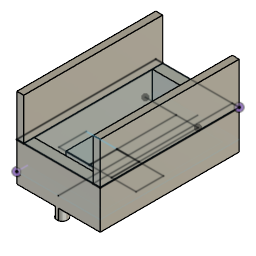
hexbug case v1 (Autodesk Fusion 360 design; units mm, degrees)
Autodesk Fusion 360 part; units mm, degrees
note: some values were not read from the file. Set by a fixed rule: which sketch regions a step uses.
sketch "Sketch1" plane through (0, 0, 0) normal (0, 0, 1) x (1, 0, 0)
  line L0 (0, 0) -> (-15.24, 0)
  line L1 (-15.24, 0) -> (-15.24, -25.4)
  line L2 (-15.24, -25.4) -> (0, -25.4)
  line L3 (0, -25.4) -> (0, 0)
  line L4 (0, 0) -> (-1.27, 0)
  line L5 (-1.27, 0) -> (-1.27, -25.4)
  line L6 (-1.27, -25.4) -> (0, -25.4)
  line L7 (0, -25.4) -> (0, 0)
  line L8 (-15.24, 0) -> (-13.97, 0)
  line L9 (-13.97, 0) -> (-13.97, -25.4)
  line L10 (-13.97, -25.4) -> (-15.24, -25.4)
  line L11 (-15.24, -25.4) -> (-15.24, 0)
  dimension "d1" = 25.4
  dimension "d2" = 15.24
  dimension "d3" = 25.4
  dimension "d4" = 1.27
  dimension "d5" = 25.4
  dimension "d6" = 1.27
  constraint horizontal L0
  constraint vertical L1
  constraint horizontal L2
  constraint vertical L3
  constraint coincident L0.start L3.end
  constraint horizontal L4
  constraint vertical L5
  constraint horizontal L6
  constraint vertical L7
  constraint horizontal L8
  constraint vertical L9
  constraint horizontal L10
  constraint vertical L11
  measures "d1" distance of L0.start L2.end
  measures "d2" distance of L0.start L0.end
  measures "d3" distance of L0.start L2.end
  measures "d4" distance of L0.start L4.end
  measures "d5" distance of L0.end L1.end
  measures "d6" distance of L0.end L8.end
extrude "Extrude1" add sketch "Sketch1" along normal blind 7.62 contours L0 L2 L3 L4 L5 L6 L7 | L0 L1 L2 L8 L9 L10 L11 makes body 1 at (0, -8.4667, 5.08) makes body 2 at (-15.24, -16.9333, 5.08)
extrude "Extrude2" add sketch "Sketch1" against normal blind 5.08 separate body makes body 3
sketch "Sketch2" plane through (0, 0, -5.08) normal (0, 0, -1) x (1, 0, 0)
  line L0 (0, 25.4) -> (-15.24, 25.4)
  line L1 (-15.24, 25.4) -> (-15.24, 0)
  line L2 (-15.24, 0) -> (0, 0)
  line L3 (0, 0) -> (0, 25.4)
  line L4 (0, 0) -> (-8.89, 0)
  line L5 (-8.89, 0) -> (-7.62, 25.4)
  line L6 (-1.143, 1.905) -> (-15.367, 1.905)
  line L7 (-15.367, 1.905) -> (-15.367, 23.495)
  line L8 (-15.367, 23.495) -> (-1.143, 23.495)
  line L9 (-1.143, 23.495) -> (-1.143, 1.905)
  line L10 (-1.143, 1.905) -> (-15.367, 23.495) construction
  line L11 (-15.367, 1.905) -> (-1.143, 23.495) construction
  point P0 (-8.255, 12.7)
  dimension "d11" = 8.89
  dimension "d12" = 21.59
  dimension "d13" = 14.224
  constraint coincident L2.end L3.start
  constraint perpendicular L1 L4
  constraint midpoint L0 L5.end
  constraint horizontal L6
  constraint perpendicular L6 L7
  constraint parallel L6 L8
  constraint parallel L7 L9
  constraint coincident L10 P0
  constraint coincident L11 P0
  constraint midpoint L5 P0
  measures "d11" distance of L2.end L4.end
  measures "d12" distance of L6.end L7.end
  measures "d13" distance of L6.start L6.end
extrude "Extrude3" cut sketch "Sketch2" against normal blind 5.08 contours L5 L6 L8 L9 | L1 L5 L6 L8 | L1 L6 L7 L8 bodies 3
sketch "Sketch3" plane through (0, 0, -5.08) normal (0, 0, -1) x (1, 0, 0)
  line L0 (-15.24, 23.495) -> (-1.143, 23.495)
  line L1 (-1.143, 23.495) -> (-1.143, 1.905)
  line L2 (-1.143, 1.905) -> (-15.24, 1.905)
  line L3 (0, 25.4) -> (-15.24, 25.4)
  line L4 (-15.24, 1.905) -> (-15.24, 0)
  line L5 (-15.24, 0) -> (0, 0)
  line L6 (0, 0) -> (0, 25.4)
  line L7 (-7.62, 0) -> (-7.62, 25.4)
  line L8 (-7.62, 12.7) -> (-9.62, 12.7)
  line L9 (-9.62, 12.7) -> (-5.62, 12.7)
  line L10 (-5.62, 12.7) -> (-5.62, 1.905)
  line L11 (-5.62, 1.905) -> (-9.62, 1.905)
  line L12 (-9.62, 1.905) -> (-9.62, 12.7)
  line L13 (-9.62, 12.7) -> (-5.62, 12.7)
  line L14 (-5.62, 12.7) -> (-5.62, 17.7)
  line L15 (-5.62, 17.7) -> (-9.62, 17.7)
  line L16 (-9.62, 17.7) -> (-9.62, 12.7)
  line L17 (-9.62, 17.7) -> (-15.24, 17.7)
  line L18 (-15.24, 17.7) -> (-15.24, 12.7)
  line L19 (-15.24, 12.7) -> (-9.62, 12.7)
  line L20 (-9.62, 12.7) -> (-9.62, 17.7)
  line L21 (-5.62, 17.7) -> (-1.143, 17.7)
  line L22 (-1.143, 17.7) -> (-1.143, 12.7)
  line L23 (-1.143, 12.7) -> (-5.62, 12.7)
  line L24 (-5.62, 12.7) -> (-5.62, 17.7)
  line L25 (-15.24, 25.4) -> (-15.24, 23.495)
  line L26 (-9.62, 1.905) -> (-15.24, 1.905)
  dimension "d16" = 2
  dimension "d17" = 4
  dimension "d18" = 5
  dimension "d19" = 4
  dimension "d32" = 5.62
  constraint midpoint L5 L7.start
  constraint midpoint L3 L7.end
  constraint midpoint L7 L8.start
  constraint perpendicular L4 L8
  constraint horizontal L9
  constraint vertical L10
  constraint horizontal L11
  constraint vertical L12
  constraint coincident L2 L10.end
  constraint horizontal L13
  constraint vertical L14
  constraint horizontal L15
  constraint vertical L16
  constraint horizontal L17
  constraint vertical L18
  constraint horizontal L19
  constraint vertical L20
  constraint horizontal L21
  constraint vertical L22
  constraint horizontal L23
  constraint vertical L24
  constraint midpoint L1 L22.end
  constraint coincident L2.end L4.start
  measures "d16" distance of L8.start L8.end
  measures "d17" distance of L10.end L11.end
  measures "d18" distance of L8.end L15.end
  measures "d19" distance of L14.end L15.end
  measures "d32" distance of L15.end L17.end
extrude "Extrude4" add sketch "Sketch3" along normal blind 2 separate body contours L7 L9 L13 L14 L15 L24 | L7 L8 L9 L13 L15 L16 L20 | L1 L14 L21 L22 L23 L24 | L2 L7 L9 L10 L11 L13 | L2 L7 L8 L9 L11 L12 L13 | L16 L17 L18 L19 L20 makes body 4
extrude "Extrude5" add 1 faces at (-5.461, -0.635, -5.08) along direction (0, 0, -1) blind 2 on bodies 3 bodies 3 4
sketch "Sketch4" plane through (0, 0, -7.08) normal (0, 0, -1) x (1, 0, 0)
  line L0 (-1.143, 17.7) -> (-15.24, 17.7)
  line L1 (-15.24, 23.495) -> (-1.143, 23.495)
  line L2 (-1.143, 23.495) -> (-1.143, 17.7)
  line L3 (-1.143, 12.7) -> (-1.143, 1.905)
  line L4 (-9.62, 1.905) -> (-15.24, 1.905)
  line L5 (-5.62, 1.905) -> (-5.62, 12.7)
  line L6 (-5.62, 12.7) -> (-1.143, 12.7)
  line L7 (0, 25.4) -> (-15.24, 25.4)
  line L8 (-15.24, 1.905) -> (-15.24, 0)
  line L9 (-15.24, 0) -> (0, 0)
  line L10 (0, 0) -> (0, 25.4)
  line L11 (-15.24, 12.7) -> (-9.62, 12.7)
  line L12 (-9.62, 12.7) -> (-9.62, 1.905)
  line L13 (-7.62, 0) -> (-7.62, 25.4)
  line L14 (-5.62, 0) -> (-5.62, 1.905)
  line L15 (-5.62, 0.9525) -> (-9.4411, 0.0417)
  line L16 (-8.1915, 23.495) -> (-7.62, 25.4)
  line L17 (-8.1915, 23.495) -> (-10.1072, 24.0697)
  line L18 (-10.1072, 24.0697) -> (-10.1072, 25.4)
  line L19 (-6.2758, 22.9203) -> (-6.2758, 25.4)
  line L20 (-6.2758, 24.1602) -> (-10.1072, 24.7348)
  circle A0 centre (-7.9057, 24.4475) radius 0.9944
  line L21 (-15.24, 17.7) -> (-15.24, 12.7)
  line L22 (-15.24, 25.4) -> (-15.24, 23.495)
  line L23 (-9.62, 1.905) -> (-5.62, 1.905)
  line L24 (-9.62, 1.905) -> (-9.62, 0)
  line L25 (-7.62, 1.905) -> (-7.62, 0)
  line L26 (-7.62, 0.9525) -> (-5.62, 0.9525)
  circle A1 centre (-7.62, 0.9525) radius 1
  line L27 (-15.24, 1.905) -> (-9.62, 1.905)
  line L28 (-5.62, 1.905) -> (-9.62, 1.905)
  line L29 (-1.143, 1.905) -> (-5.62, 1.905)
  dimension "d25" = 2
  dimension "d26" = 2
  dimension "d31" = 2
  constraint midpoint L9 L13.start
  constraint midpoint L7 L13.end
  constraint coincident L9 L14.start
  constraint coincident L5.start L14.end
  constraint perpendicular L4 L14
  constraint midpoint L14 L15.start
  constraint midpoint L1 L16.start
  constraint perpendicular L16 L17
  constraint coincident L7 L18.end
  constraint perpendicular L7 L18
  constraint coincident L7 L19.end
  constraint perpendicular L7 L19
  constraint midpoint L19 L20.start
  constraint midpoint L18 L20.end
  constraint midpoint L16 A0.centre
  constraint coincident L13.end A0
  constraint coincident L4.start L12.end
  constraint coincident L14 L5.start
  constraint perpendicular L14 L23
  constraint coincident L9 L24.end
  constraint perpendicular L9 L24
  constraint coincident L13 L25.start
  constraint coincident L4 L25.start
  constraint midpoint L25 L26.start
  constraint coincident L14 L15.start
  constraint perpendicular L14 L26
  constraint coincident L26.start A1.centre
  constraint coincident L4.end L8.start
  constraint coincident L24 L4.start
  constraint coincident L4 L12.end
  constraint coincident L4 L5.start
  measures "d25" distance of L16.start L17.end
  measures "d26" distance of L16.start L19.start
  measures "d31" diameter of A1
extrude "Extrude8" add sketch "Sketch1" against normal blind 5 separate body contours L0 L1 L2 L8 L9 L10 L11 makes body 5
extrude "Extrude9" add 1 faces at (-14.8167, -8.4667, -5) along direction (0, 0, -1) blind 2 on bodies 5 bodies 3 5
extrude "Extrude10" add 2 faces at (-14.8167, -19.6317, -7) (-14.8167, -9.1017, -7) along direction (0, 0, -1) blind 0.08 on bodies 3 bodies 3
extrude "Extrude11" add sketch "Sketch4" along normal blind 2 contours L1 L13 L16 L20 | L13 L20 A0 | L13 L23 L25 L26 A1 L28 | L13 L15 L23 L25 A1 L28 | L16 L20 A0 | L13 L16 L20 | L13 L20 A0 | L13 L15 L25 L26 A1 | L9 L13 L15 L25 A1 | L7 L16 L20 A0 | L9 L13 L15 L25 A1 bodies 3
extrude "Extrude6" [rolled back] along distance 2 taper angle 0
extrude "Extrude7" [rolled back] along distance -5 taper angle 0
extrude "Extrude12" [rolled back] along distance 4 taper angle 0
extrude "Extrude13" [rolled back] along distance 2 taper angle 0
sketch "Sketch5" plane through (0, 0, 0) normal (0, 1, 0) x (-1, 0, 0)
  line L0 (7.3155, -7.08) -> (7.9245, -7.08)
  line L1 (7.9245, -7.08) -> (15.24, -7.08)
  line L2 (15.24, -7.08) -> (15.24, 7.62)
  line L3 (15.24, 7.62) -> (13.97, 7.62)
  line L4 (13.97, 7.62) -> (13.97, 0)
  line L5 (13.97, 0) -> (0, 0)
  line L6 (0, 0) -> (0, -7.08)
  line L7 (0, -7.08) -> (7.3155, -7.08)
  line L8 (0, 0) -> (15.24, 0)
  line L9 (7.62, -7.08) -> (7.62, 0)
  line L10 (7.62, -7.08) -> (7.62, -5.08)
  line L11 (0, 0) -> (1.25, 0)
  line L12 (15.24, 0) -> (13.99, 0)
  line L13 (7.62, -5.08) -> (1.25, 0)
  line L14 (13.97, 0) -> (7.62, -5.08)
  line L15 (4.435, -2.54) -> (4.435, -5.08)
  arc A0 (1.25, 0) -> (7.62, -5.08) centre (9.1392, 3.3588) ccw
  line L16 (10.795, -2.54) -> (10.795, -5.08)
  arc A1 (7.62, -5.08) -> (13.97, 0) centre (6.096, 3.3338) ccw
  dimension "d45" = 2
  dimension "d46" = 1.25
  dimension "d47" = 1.25
  dimension "d48" = 2.54
  dimension "d49" = 2.54
  constraint coincident L5.end L6.start
  constraint coincident L2 L8.end
  constraint perpendicular L2 L8
  constraint midpoint L0 L9.start
  constraint midpoint L8 L9.end
  constraint perpendicular L8 L10
  constraint perpendicular L6 L11
  constraint perpendicular L2 L12
  constraint coincident L4.end L5.start
  constraint midpoint L13 L15.start
  constraint parallel L10 L15
  constraint midpoint L14 L16.start
  constraint vertical L16
  measures "d45" distance of L9.start L10.end
  measures "d46" distance of L5.end L11.end
  measures "d47" distance of L8.end L12.end
  measures "d48" distance of L15.start L15.end
  measures "d49" distance of L16.start L16.end
extrude "Extrude14" [rolled back] along distance -25.4 taper angle 0
